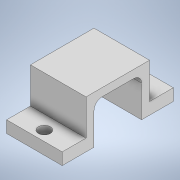
# Autodesk Inventor part: мотор
Saved by Autodesk Inventor 2020 (Build 240168000, 168)
## iProperties
Created: 2024-03-26
Part Number: мотор
Material: Типовые
Document SubType Name: Modeling
Designer: user
Density: 1 g/cm^3
Appearance: По умолчанию
Author: user
Autodesk Inventor part; units mm, degrees
ref_plane "YZ Plane" through (0, 0, 0) normal (1, 0, 0) x (0, 1, 0)
ref_plane "XZ Plane" through (0, 0, 0) normal (0, 1, 0) x (-1, 0, 0)
ref_plane "XY Plane" through (0, 0, 0) normal (0, 0, 1) x (1, 0, 0)
sketch "Эскиз1" plane through (0, 0, 0) normal (0, 1, 0) x (-1, 0, 0)
  line L0 (-7, 6) -> (7, 6)
  line L1 (7, 6) -> (7, 14)
  line L2 (7, 14) -> (-7, 14)
  line L3 (-7, 14) -> (-7, 6)
  line L4 (9.7319, 0) -> (-12.3676, 0)
  line L5 (-7, -6) -> (7, -6)
  line L6 (7, -6) -> (7, -14)
  line L7 (7, -14) -> (-7, -14)
  line L8 (-7, -14) -> (-7, -6)
  circle A0 centre (0, 11.5) radius 1.5
  circle A1 centre (0, -11.5) radius 1.5
  point P0 (0, 0)
  dimension "d0" = 14
  dimension "d1" = 8
  dimension "d2" = 14
  dimension "d3" = 7
  dimension "d4" = 3
  dimension "d5" = 11.5
  dimension "d6" = 7
  constraints: 18 end point, 5 symmetric about line, 2 centre point, 2 horizontal, 2 parallel, 1 perpendicular, 1 other
  measures "d0" distance of L2.end L1.end
  measures "d1" distance of L1.end L0.end
  measures "d2" distance from line of L2 point (0, 0)
  measures "d3" distance from line of L1 point (0, 0)
  measures "d4" diameter of A0
  measures "d5" distance of point (0, 0) A0.centre
  measures "d6" distance from line of L1 A0.centre
extrude "Выдавливание1" add sketch "Эскиз1" along normal blind 3
sketch "Эскиз2" plane through (0, 3, 0) normal (0, 1, 0) x (1, 0, 0)
  line L0 (7, -6) -> (-7, -6) projected
  line L1 (7, -14) -> (7, -6) projected
  line L2 (-7, -6) -> (7, -6)
  line L3 (7, -6) -> (7, -8)
  line L4 (7, -8) -> (-7, -8)
  line L5 (-7, -8) -> (-7, -6)
  line L6 (-8.7182, 0) -> (11.1511, 0)
  line L7 (7, 6) -> (-7, 6)
  line L8 (7, 14) -> (7, 6)
  line L9 (7, 8) -> (-7, 8)
  line L10 (-7, 8) -> (-7, 6)
  point P0 (0, 0)
  dimension "d9" = 2
  constraints: 18 end point, 5 symmetric about line, 2 horizontal, 2 parallel, 2 point on line, 1 perpendicular
  measures "d9" distance of L2.end L3.end
extrude "Выдавливание2" add sketch "Эскиз2" along normal blind 9
sketch "Эскиз3" plane through (-7, 3, 8) normal (0, 0, 1) x (1, 0, 0)
  line L0 (0, -3) -> (0, 9) projected
  line L1 (0, 9) -> (14, 9)
  line L2 (14, 9) -> (14, 7)
  line L3 (14, 7) -> (0, 7)
  line L4 (0, 7) -> (0, 9)
  point P0 (7, -3)
  dimension "d12" = 2
  constraints: 8 end point, 2 parallel, 1 horizontal, 1 perpendicular
  measures "d12" distance of L1.end L2.end
extrude "Выдавливание3" add sketch "Эскиз3" against normal through all
sketch "Эскиз4" plane through (7, 0, 14) normal (1, 0, 0) x (0, 0, -1)
  line L0 (8, 10) -> (20, 10) projected
  line L1 (8, 0) -> (8, 10) projected
  arc A0 (10, 10) -> (8, 8) centre (10, 8) ccw
  line L2 (8, 8) -> (10, 10) construction
  line L3 (8, 8) -> (10.8284, 8) construction
  line L4 (14, 0) -> (14, 12)
  line L5 (22, 12) -> (6, 12) projected
  arc A1 (20, 8) -> (18, 10) centre (18, 8) ccw
  line L6 (20, 0) -> (20, 10) projected
  line L7 (22, 3) -> (22, 12) projected
  line L8 (6, 12) -> (22, 12) projected
  line L9 (6, 3) -> (6, 12) projected
  line L10 (0, 3) -> (6, 3) projected
  line L11 (0, 0) -> (0, 3) projected
  line L12 (0, 0) -> (8, 0) projected
  line L13 (8, 0) -> (8, 10) projected
  line L14 (8, 10) -> (20, 10) projected
  line L15 (20, 0) -> (20, 10) projected
  line L16 (20, 0) -> (28, 0) projected
  line L17 (28, 0) -> (28, 3) projected
  line L18 (22, 3) -> (28, 3) projected
  point P0 (18, 10)
  dimension "d15" = 45
  constraints: 6 end point, 4 point on circle, 3 symmetric about line, 2 centre point, 2 point on line, 1 equal length, 1 horizontal, 1 midpoint, 1 tangent, 1 other
  measures "d15" angle of L3 L2
extrude "Выдавливание4" add sketch "Эскиз4" against normal blind 2 contours L0 A0 L1 | L0 L6 A1
sketch "Эскиз5" plane through (-7, 0, -14) normal (-1, 0, 0) x (0, 0, 1)
  arc A0 (10, 10) -> (8, 8) centre (10, 8) ccw projected
  line L0 (8, 10) -> (10, 10) projected
  line L1 (8, 8) -> (8, 10) projected
  line L2 (20, 10) -> (20, 8) projected
  line L3 (18, 10) -> (20, 10) projected
  arc A1 (20, 8) -> (18, 10) centre (18, 8) ccw projected
  point P0 (14, 0)
extrude "Выдавливание5" add sketch "Эскиз5" against normal blind 2
